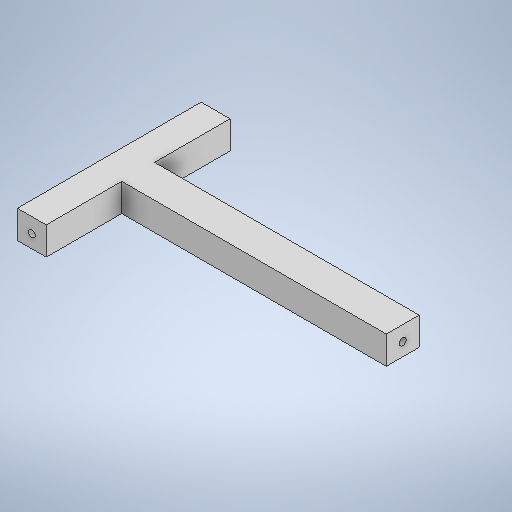
# Autodesk Inventor part: T
Saved by Autodesk Inventor 2025.3 (Build 293356000, 356)
## iProperties
Created: 2026-04-07
Part Number: T
Material: Generic
Document SubType Name: Modeling
Designer: ksawe
Density: 1 g/cm^3
Appearance: Default
Author: ksawe
Autodesk Inventor part; units mm, degrees
ref_plane "YZ Plane" through (0, 0, 0) normal (1, 0, 0) x (0, 1, 0)
ref_plane "XZ Plane" through (0, 0, 0) normal (0, 1, 0) x (-1, 0, 0)
ref_plane "XY Plane" through (0, 0, 0) normal (0, 0, 1) x (1, 0, 0)
sketch "Sketch1" plane through (0, 0, 0) normal (0, 1, 0) x (-1, 0, 0)
  line L0 (-52.0419, 20) -> (-52.0419, -20)
  line L1 (52.0419, 20) -> (-52.0419, -20) construction
  line L2 (-52.0419, 20) -> (52.0419, -20) construction
  line L3 (305.5497, 112) -> (270.3665, 112)
  line L4 (270.3665, -112) -> (305.5497, -112)
  line L5 (305.5497, -112) -> (305.5497, 112)
  line L6 (305.5497, 112) -> (270.3665, -112) construction
  line L7 (270.3665, 112) -> (305.5497, -112) construction
  line L8 (270.3665, 20) -> (-52.0419, 20)
  line L9 (270.3665, 112) -> (270.3665, 20)
  line L10 (270.3665, -20) -> (270.3665, -112)
  line L11 (-52.0419, -20) -> (270.3665, -20)
  point P0 (0, 0)
  point P1 (287.9581, 0)
  point P2 (-52.0419, 0)
  dimension "d17" = 224
  dimension "d19" = 40
  dimension "d20" = 340
  constraints: 24 end point, 5 midpoint, 4 parallel, 3 perpendicular, 2 horizontal, 2 horizontal alignment
  measures "d17" distance of L4.end L3.start
  measures "d19" distance between parallel lines of L11 L8
  measures "d20" distance from line of L0 point (287.958, 0)
extrude "Extrusion1" add sketch "Sketch1" along normal blind 34
sketch "Sketch2" plane through (-305.5497, 0, 112) normal (0, 0, 1) x (1, 0, 0)
  circle A0 centre (17.5916, 16) radius 4.25
  line L0 (0, 0) -> (35.1832, 0) projected
  line L1 (0, 0) -> (0, 34) projected
  point P0 (305.5497, 0)
  point P1 (17.5916, 0)
  dimension "d2" = 8.5
  dimension "d3" = 16
  constraints: 1 centre point, 1 midpoint, 1 vertical alignment
  measures "d2" diameter of A0
  measures "d3" distance from line of L0 A0.centre
sketch "Sketch3" plane through (52.0419, 0, 20) normal (1, 0, 0) x (0, 0, -1)
  circle A0 centre (20, 16) radius 4.25
  line L0 (0, 0) -> (40, 0) projected
  line L1 (40, 0) -> (40, 34) projected
  point P0 (20, 0)
  point P1 (20, 0)
  dimension "d4" = 8.5
  dimension "d5" = 16
  constraints: 1 centre point, 1 midpoint, 1 vertical alignment
  measures "d4" diameter of A0
  measures "d5" distance from line of L0 A0.centre
sketch "Sketch4" plane through (-270.3665, 0, -112) normal (0, 0, -1) x (-1, 0, 0)
  circle A0 centre (17.5916, 16) radius 4.25
  line L0 (0, 0) -> (35.1832, 0) projected
  line L1 (0, 0) -> (0, 34) projected
  point P0 (-270.3665, 0)
  point P1 (17.5916, 0)
  dimension "d6" = 8.5
  dimension "d7" = 16
  constraints: 1 centre point, 1 midpoint, 1 vertical alignment
  measures "d6" diameter of A0
  measures "d7" distance from line of L0 A0.centre
extrude "Extrusion2" cut sketch "Sketch4" against normal blind 10
extrude "Extrusion3" cut sketch "Sketch2" against normal blind 10
extrude "Extrusion4" cut sketch "Sketch3" against normal blind 10
body "Solid1"
